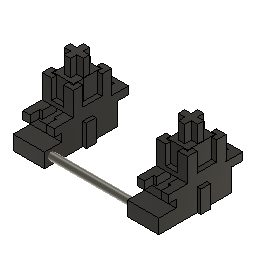
MX Cherry-style Stabilizer v10 (Autodesk Fusion 360 design; units mm, degrees)
Autodesk Fusion 360 part; units mm, degrees
note: some values were not read from the file. Chosen so that the rebuilt part matches the saved one: which bodies a step acts on; which face or edge a step refers to. Set by a fixed rule: which sketch regions a step uses.
sketch "Post Hole" plane through (0, 0, 0) normal (0, 0, 1) x (1, 0, 0)
  line L0 (-11.9, 5.93) -> (-7.7, 5.93)
  line L1 (-11.9, -7.57) -> (-10.4, -7.57)
  line L2 (1.75, 0) -> (22.5, 0)
  line L3 (-8.575, 2.3) -> (-7.7, 2.3)
  line L4 (-7.7, -0.5) -> (-7.7, 7.93)
  line L5 (-8.575, -0.5) -> (-7.7, -0.5)
  line L6 (-8.575, -0.5) -> (-8.575, -9.77)
  line L7 (-10.4, -6.77) -> (-8.575, -6.77)
  line L8 (-10.4, -8.27) -> (-10.4, -6.77)
  line L9 (-8.575, -9.77) -> (-11.9, -9.77)
  line L10 (-11.9, 9.93) -> (-8.575, 9.93)
  line L11 (-8.575, 9.93) -> (-8.575, 2.3)
  line L12 (-10.4, -8.27) -> (-11.9, -8.27)
  line L13 (-7.7, 7.93) -> (-11.9, 7.93)
  line L14 (-11.9, 11) -> (-11.9, -15.5609)
  line L15 (-10, -20) -> (13.8, -20)
  line L16 (-11.9, -7.57) -> (-13.4, -7.57)
  line L17 (-15.225, 9.93) -> (-15.225, 2.3)
  line L18 (-13.4, -8.27) -> (-13.4, -6.77)
  line L19 (-16.1, -0.5) -> (-16.1, 7.93)
  line L20 (-16.1, 7.93) -> (-11.9, 7.93)
  line L21 (-15.225, -0.5) -> (-16.1, -0.5)
  line L22 (-11.9, 5.93) -> (-16.1, 5.93)
  line L23 (-13.4, -6.77) -> (-15.225, -6.77)
  line L24 (-11.9, 9.93) -> (-15.225, 9.93)
  line L25 (-15.225, -0.5) -> (-15.225, -9.77)
  line L26 (-13.4, -8.27) -> (-11.9, -8.27)
  line L27 (-15.225, -9.77) -> (-11.9, -9.77)
  line L28 (-15.225, 2.3) -> (-16.1, 2.3)
  point P0 (-11.9, 11)
  dimension "d3" = 13.5
  dimension "d10" = 2
  dimension "d11" = 3
  dimension "d13" = 4
  dimension "d75" = 1.5
  dimension "d78" = 2.8
  dimension "d79" = 0.875
  dimension "d80" = 4.2
  dimension "d82" = 0.8
  dimension "d83" = 6.77
  dimension "d84" = 0.7
  dimension "d85" = 0.5
  dimension "ParameterA" = 23.8
  dimension "d87" = 11.9
  constraint coincident L14 L12.end
  constraint coincident L14 L1.start
  constraint coincident L14 L9.end
  constraint coincident L14 L0.start
  constraint coincident L14 L13.end
  constraint coincident L14 L10.start
  constraint coincident L4 L0.end
  constraint coincident L3.end L4
  constraint coincident L7.end L6
  constraint coincident L1.end L8
  constraint vertical L4
  constraint collinear L6 L11
  constraint horizontal L15
  constraint symmetric L1.end L14 L16.end
  constraint symmetric L3.start L14 L17.end
  constraint symmetric L3.end L14 L28.end
  constraint symmetric L4.start L14 L19.start
  constraint symmetric L5.start L14 L21.start
  constraint symmetric L7.end L14 L23.end
  constraint symmetric L7.start L14 L18.end
  constraint symmetric L6.end L14 L25.end
  constraint symmetric L10.end L14 L17.start
  constraint symmetric L8.start L14 L18.start
  constraint symmetric L4.end L14 L19.end
  constraint symmetric P0 L14 L14.start
  constraint symmetric L14 L12.end L26.end
  constraint symmetric L14 L1.start L16.start
  constraint symmetric L14 L9.end L27.end
  constraint symmetric L14 L13.end L20.end
  constraint symmetric L14 L10.start L24.start
  constraint symmetric L14 L0.start L22.start
  constraint symmetric L14 L0.end L22.end
  measures "d3" distance of L0 L1
  measures "d10" distance of L0 L13
  measures "d11" distance of L7 L9
  measures "d13" distance of L0 L10
  measures "d75" distance of L8 L14
  measures "d78" distance of L3 L5
  measures "d79" distance of L4 L6
  measures "d80" distance of L4 L14
  measures "d82" distance of L1 L7
  measures "d83" distance of L2 L7
  measures "d84" distance of L1 L12
  measures "d85" distance of L2 L5
  measures "ParameterA" distance of L15.start L15.end
  measures "d87" distance of origin L14
ref_plane "WorkPlane1" through (0, 0, -1.6) normal (0, 0, 1) x (1, 0, 0)
extrude "Extrude1" add sketch "Post Hole" along normal blind 10 contours L0 L11 L13 L14 | L14 L17 L20 L22 | L0 L1 L3 L4 L5 L6 L7 L8 L11 L14 | L14 L16 L17 L18 L19 L21 L22 L23 L25 L28 | L0 L4 L11 L13 | L0 L3 L4 L11 | L1 L8 L12 L14 | L14 L16 L18 L26 | L17 L19 L20 L22 | L17 L19 L22 L28 | L6 L7 L8 L9 L12 L14 | L14 L18 L23 L25 L26 L27 makes body 1
extrude "Extrude2" add sketch "Post Hole" against normal up to surface (1.6 mm away) separate body contours L0 L1 L3 L4 L5 L6 L7 L8 L11 L14 | L14 L16 L17 L18 L19 L21 L22 L23 L25 L28 makes body 2
extrude "Extrude3" add sketch "Post Hole" against normal blind 10 from surface at -1.6 separate body contours L0 L11 L13 L14 | L14 L17 L20 L22 | L0 L1 L3 L4 L5 L6 L7 L8 L11 L14 | L14 L16 L17 L18 L19 L21 L22 L23 L25 L28 | L10 L11 L13 L14 | L14 L17 L20 L24 | L1 L8 L12 L14 | L14 L16 L18 L26 makes body 3
sketch "Placeholder over Plate" plane through (0, 0, 0) normal (0, 0, 1) x (1, 0, 0)
  line L0 (1.75, 0) -> (22.5, 0)
  line L1 (-11.9, -7.5) -> (-8.65, -7.5)
  line L2 (20, 0) -> (2.5, 0)
  line L3 (-8.65, -4) -> (-11.9, -4)
  line L4 (-10.65, 4) -> (-10.65, 3)
  line L5 (-11.9, 3) -> (-9.65, 3)
  line L6 (-9.65, 2) -> (-8.65, 2)
  line L7 (-10.65, -3) -> (-9.65, -3)
  line L8 (-9.65, -3) -> (-9.65, 3)
  line L9 (-9.65, -2) -> (-8.65, -2)
  line L10 (-10.15, 8) -> (-10.15, 6)
  line L11 (-10.15, 6) -> (-10.65, 6)
  line L12 (-10.65, 6) -> (-10.65, 4)
  line L13 (-10.65, -3) -> (-10.65, -6.5)
  line L14 (-10.65, -6.5) -> (-11.9, -6.5)
  line L15 (-11.9, -5.2) -> (-8.65, -5.2)
  line L16 (-8.65, 0) -> (-7.9, 0)
  line L17 (-7.9, 0) -> (-7.9, 2)
  line L18 (-7.9, 2) -> (-8.65, 2)
  line L19 (-8.65, -7.5) -> (-8.65, 10)
  line L20 (-8.65, 10) -> (-11.9, 10)
  line L21 (-11.9, -10) -> (-11.9, 12)
  line L22 (-8.65, 4) -> (-11.9, 4)
  line L23 (-11.9, 6.4) -> (-8.65, 6.4)
  line L24 (-11.9, 8) -> (-8.65, 8)
  line L25 (-11.9, 6.4) -> (-15.15, 6.4)
  line L26 (-13.65, 6) -> (-13.15, 6)
  line L27 (-11.9, 3) -> (-14.15, 3)
  line L28 (-13.15, 4) -> (-13.15, 3)
  line L29 (-13.65, 8) -> (-13.65, 6)
  line L30 (-15.15, 10) -> (-11.9, 10)
  line L31 (-13.15, 6) -> (-13.15, 4)
  line L32 (-15.15, -7.5) -> (-15.15, 10)
  line L33 (-13.15, -6.5) -> (-11.9, -6.5)
  line L34 (-14.15, 2) -> (-15.15, 2)
  line L35 (-11.9, -5.2) -> (-15.15, -5.2)
  line L36 (-13.15, -3) -> (-13.15, -6.5)
  line L37 (-15.15, 0) -> (-15.9, 0)
  line L38 (-15.9, 0) -> (-15.9, 2)
  line L39 (-15.15, 4) -> (-11.9, 4)
  line L40 (-14.15, -2) -> (-15.15, -2)
  line L41 (-11.9, -7.5) -> (-15.15, -7.5)
  line L42 (-15.9, 2) -> (-15.15, 2)
  line L43 (-14.15, -3) -> (-14.15, 3)
  line L44 (-15.15, -4) -> (-11.9, -4)
  line L45 (-13.15, -3) -> (-14.15, -3)
  line L46 (-11.9, 8) -> (-15.15, 8)
  line L47 (-7.15, -9.5) -> (-16.65, -9.5)
  line L48 (-16.65, -9.5) -> (-16.65, 9.5)
  line L49 (-16.65, 9.5) -> (-7.15, 9.5)
  line L50 (-7.15, 9.5) -> (-7.15, -9.5)
  line L51 (-7.15, -9.5) -> (-16.65, 9.5) construction
  line L52 (-16.65, -9.5) -> (-7.15, 9.5) construction
  point P0 (-11.9, 12)
  point P1 (-11.9, -10)
  point P2 (-11.9, 0)
  dimension "d23" = 15.5
  dimension "d25" = 8
  dimension "d26" = 1
  dimension "d27" = 1
  dimension "d29" = 2
  dimension "d30" = 1.5
  dimension "d32" = 1
  dimension "d57" = 1.2
  dimension "d59" = 6
  dimension "d88" = 11.9
  dimension "d89" = 4
  dimension "d90" = 3.25
  dimension "d91" = 2
  dimension "d92" = 1.25
  dimension "d93" = 8
  dimension "d94" = 2.4
  dimension "d133" = 19
  dimension "d134" = 9.5
  constraint coincident L22.start L19
  constraint symmetric L22.start L2 L3.start
  constraint coincident L4.start L22
  constraint perpendicular L4 L22
  constraint perpendicular L4 L5
  constraint perpendicular L5 L8
  constraint coincident L6.end L19
  constraint perpendicular L6 L19
  constraint symmetric L2 L4.end L7.start
  constraint symmetric L2 L5.end L7.end
  constraint symmetric L2 L6.start L9.start
  constraint symmetric L2 L6.end L9.end
  constraint perpendicular L10 L11
  constraint perpendicular L11 L12
  constraint perpendicular L3 L13
  constraint perpendicular L13 L14
  constraint coincident L15.end L19
  constraint perpendicular L15 L19
  constraint coincident L23.end L19
  constraint coincident L16.start L19
  constraint perpendicular L16 L19
  constraint perpendicular L0 L17
  constraint perpendicular L19 L20
  constraint collinear L0 L16
  constraint perpendicular L17 L18
  constraint coincident L21 L1.start
  constraint coincident L21 L15.start
  constraint coincident L21 L3.end
  constraint coincident L21 L5.start
  constraint coincident L21 L22.end
  constraint coincident L21 L23.start
  constraint coincident L21 L24.start
  constraint coincident L24.end L19
  constraint coincident L4.end L5
  constraint coincident L6.start L8
  constraint coincident L14.end L21
  constraint coincident L10.start L24
  constraint symmetric L24.end L21 L46.end
  constraint symmetric L1.end L21 L32.start
  constraint symmetric L22.start L21 L39.start
  constraint symmetric L3.start L21 L44.start
  constraint symmetric L4.start L21 L28.start
  constraint symmetric L4.end L21 L28.end
  constraint symmetric L5.end L21 L27.end
  constraint symmetric L6.start L21 L34.start
  constraint symmetric L6.end L21 L34.end
  constraint symmetric L7.start L21 L36.start
  constraint symmetric L7.end L21 L43.start
  constraint symmetric L9.start L21 L40.start
  constraint symmetric L9.end L21 L40.end
  constraint symmetric L10.start L21 L29.start
  constraint symmetric L10.end L21 L26.start
  constraint symmetric L11.end L21 L26.end
  constraint symmetric L13.end L21 L33.start
  constraint symmetric L14.end L21 L33.end
  constraint symmetric L15.end L21 L35.end
  constraint symmetric L23.end L21 L25.end
  constraint symmetric L16.start L21 L37.start
  constraint symmetric L16.end L21 L37.end
  constraint symmetric L17.end L21 L38.end
  constraint symmetric L19.end L21 L30.start
  constraint symmetric L20.end L21 L30.end
  constraint symmetric P1 L21 L21.start
  constraint symmetric P0 L21 L21.end
  constraint symmetric L21 L1.start L41.start
  constraint symmetric L21 L15.start L35.start
  constraint symmetric L21 L3.end L44.end
  constraint symmetric L21 L5.start L27.start
  constraint symmetric L21 L22.end L39.end
  constraint symmetric L21 L23.start L25.start
  constraint symmetric L21 L24.start L46.start
  constraint horizontal L47
  constraint perpendicular L47 L48
  constraint parallel L47 L49
  constraint parallel L48 L50
  constraint coincident L51 P2
  constraint coincident L52 P2
  constraint coincident L21 P2
  constraint coincident L2 P2
  measures "d23" distance of L24.end L1.end
  measures "d25" distance of L3 L22
  measures "d26" distance of L5 L22
  measures "d27" distance of L8 L19
  measures "d29" distance of L6 L22
  measures "d30" distance of L10 L19
  measures "d32" distance of L1 L14
  measures "d57" distance of L3 L15
  measures "d59" distance of L20 L22
  measures "d88" distance of origin L21
  measures "d89" distance of L17 L21
  measures "d90" distance of L19 L21
  measures "d91" distance of L11 L24
  measures "d92" distance of L12 L21
  measures "d93" distance of origin L24
  measures "d94" distance of L22 L23
  measures "d133" distance of L47.end L48.end
  measures "d134" distance of L47.start L47.end
extrude "Extrude4" add sketch "Placeholder over Plate" along normal blind 1.6 separate body contours L1 L13 L14 L15 L19 L21 | L21 L32 L33 L35 L36 L41 | L3 L13 L15 L19 | L32 L35 L36 L44 | L10 L19 L23 L24 | L25 L29 L32 L46 | L10 L11 L12 L19 L22 L23 | L25 L26 L29 L31 L32 L39 makes body 4 at (-9.15, 6, 0) makes body 5 at (-14.65, 6, 0) makes body 6 at (-9.3167, -6, 0)
extrude "Extrude5" add sketch "Placeholder over Plate" along normal blind 6.5 contours L3 L7 L8 L9 L13 L19 | L32 L36 L40 L43 L44 L45 | L4 L5 L6 L8 L19 L22 | L27 L28 L32 L34 L39 L43 bodies 6 4 5
extrude "Extrude6" add sketch "Placeholder over Plate" along normal blind 2.5 contours L6 L8 L9 L19 | L32 L34 L40 L43 bodies 6 4 5
extrude "Extrude7" add sketch "Placeholder over Plate" along normal blind 0.9 from surface at 1.6 contours L4 L5 L21 L22 | L21 L27 L28 L39 | L4 L5 L6 L8 L19 L22 bodies 6
sketch "Placeholder Stem" plane through (0, 0, 6.5) normal (0, 0, 1) x (-1, 0, 0)
  line L0 (11.9, -4) -> (11.9, 0)
  line L1 (11.9, 0) -> (8.4, 0)
  line L2 (11.9, -2.8) -> (9.8, -2.8)
  line L3 (9.8, -2.8) -> (9.8, 0)
  line L4 (11.9, -0.65) -> (9.9, -0.65)
  line L5 (9.9, -0.65) -> (9.9, 0)
  line L6 (-1.75, 0) -> (-22.5, 0)
  line L7 (11.9, -2) -> (11.25, -2)
  line L8 (11.25, -2) -> (11.25, 0)
  line L9 (11.9, -0.65) -> (13.9, -0.65)
  line L10 (12.55, -2) -> (12.55, 0)
  line L11 (11.9, -2.8) -> (14, -2.8)
  line L12 (14, -2.8) -> (14, 0)
  line L13 (13.9, -0.65) -> (13.9, 0)
  line L14 (11.9, -2) -> (12.55, -2)
  line L15 (13.9, 0.65) -> (13.9, 0)
  line L16 (11.9, 2.8) -> (14, 2.8)
  line L17 (9.9, 0.65) -> (9.9, 0)
  line L18 (11.9, 2) -> (11.25, 2)
  line L19 (11.25, 2) -> (11.25, 0)
  line L20 (11.9, 2.8) -> (9.8, 2.8)
  line L21 (12.55, 2) -> (12.55, 0)
  line L22 (11.9, 0.65) -> (9.9, 0.65)
  line L23 (11.9, 0.65) -> (13.9, 0.65)
  line L24 (14, 2.8) -> (14, 0)
  line L25 (9.8, 2.8) -> (9.8, 0)
  line L26 (11.9, 2) -> (12.55, 2)
  point P0 (11.9, 0)
  point P1 (11.9, 0)
  point P2 (11.9, 0)
  dimension "d95" = 2.1
  dimension "d96" = 2.8
  dimension "d97" = 11.9
  dimension "d98" = 0.65
  dimension "d99" = 2
  dimension "d100" = 0.65
  dimension "d101" = 2
  constraint vertical L0
  constraint perpendicular L0 L1
  constraint coincident L0 L2.start
  constraint perpendicular L0 L2
  constraint coincident L1 L3.end
  constraint perpendicular L1 L3
  constraint coincident L0 L4.start
  constraint perpendicular L0 L4
  constraint coincident L1 L5.end
  constraint perpendicular L1 L5
  constraint collinear L1 L6
  constraint coincident L0 L7.start
  constraint perpendicular L0 L7
  constraint coincident L1 L8.end
  constraint perpendicular L1 L8
  constraint symmetric P1 L0 P0
  constraint symmetric L0 L2.start L11.start
  constraint symmetric L0 L2.end L11.end
  constraint symmetric L0 L3.end L12.end
  constraint symmetric L0 L4.start L9.start
  constraint symmetric L0 L4.end L9.end
  constraint symmetric L0 L5.end L13.end
  constraint symmetric L0 L7.start L14.start
  constraint symmetric L0 L7.end L10.start
  constraint symmetric L0 L8.end L10.end
  constraint symmetric P1 L1 P0
  constraint symmetric L1 L2.start L16.start
  constraint symmetric L1 L2.end L20.end
  constraint symmetric L1 L3.end L25.end
  constraint symmetric L1 L4.start L22.start
  constraint symmetric L1 L4.end L17.start
  constraint symmetric L1 L5.end L17.end
  constraint symmetric L1 L7.start L18.start
  constraint symmetric L1 L7.end L18.end
  constraint symmetric L1 L8.end L19.end
  constraint symmetric L1 P2 P1
  constraint symmetric L1 L10.start L21.start
  constraint symmetric L1 L10.end L21.end
  constraint symmetric L1 L11.end L16.end
  constraint symmetric L1 L9.end L15.start
  constraint symmetric L1 L12.end L24.end
  constraint symmetric L1 L13.end L15.end
  measures "d95" distance of L0 L3
  measures "d96" distance of L1 L2
  measures "d97" distance of origin L0
  measures "d98" distance of L1 L4
  measures "d99" distance of L0 L5
  measures "d100" distance of L0 L8
  measures "d101" distance of L1 L7
extrude "Extrude8" add sketch "Placeholder Stem" against normal blind 6 separate body contours L0 L1 L2 L3 L4 L5 L7 L8 | L0 L1 L9 L10 L11 L12 L13 L14 L15 L16 L17 L18 L19 L20 L21 L22 L23 L24 L25 L26 makes body 7
extrude "Extrude9" add sketch "Placeholder Stem" along normal blind 3.5 separate body contours L0 L4 L7 L8 | L0 L9 L10 L14 | L0 L1 L4 L8 | L0 L1 L9 L10 L19 L21 L22 L23 | L1 L4 L5 L8 | L9 L10 L13 L15 L21 L23 | L1 L17 L19 L22 | L18 L19 L21 L22 L23 L26 makes body 8
extrude "Extrude10" add sketch "Placeholder over Plate" against normal blind 1.6 separate body contours L3 L13 L15 L19 | L3 L13 L15 L21 | L21 L35 L36 L44 | L32 L35 L36 L44 | L3 L7 L8 L9 L13 L19 | L3 L5 L7 L8 L13 L21 | L21 L27 L36 L43 L44 L45 | L32 L36 L40 L43 L44 L45 | L6 L8 L9 L19 | L4 L5 L21 L22 | L21 L27 L28 L39 | L32 L34 L40 L43 | L16 L17 L18 L19 | L4 L5 L6 L8 L19 L22 | L21 L25 L26 L29 L31 L39 | L10 L11 L12 L21 L22 L23 | L27 L28 L32 L34 L39 L43 | L32 L37 L38 L42 | L10 L11 L12 L19 L22 L23 | L25 L26 L29 L31 L32 L39 makes body 9
extrude "Extrude11" add sketch "Placeholder over Plate" against normal blind 3 from surface at -1.6 separate body contours L13 L14 L15 L21 | L21 L33 L35 L36 | L3 L13 L15 L19 | L3 L13 L15 L21 | L21 L35 L36 L44 | L32 L35 L36 L44 | L3 L7 L8 L9 L13 L19 | L3 L5 L7 L8 L13 L21 | L21 L27 L36 L43 L44 L45 | L32 L36 L40 L43 L44 L45 | L6 L8 L9 L19 | L4 L5 L21 L22 | L21 L27 L28 L39 | L19 L20 L21 L49 | L19 L21 L24 L49 | L21 L32 L46 L49 | L21 L30 L32 L49 | L32 L34 L40 L43 | L16 L17 L18 L19 | L4 L5 L6 L8 L19 L22 | L21 L25 L26 L29 L31 L39 | L10 L11 L12 L21 L22 L23 | L27 L28 L32 L34 L39 L43 | L10 L19 L23 L24 | L25 L29 L32 L46 | L32 L37 L38 L42 | L10 L11 L12 L19 L22 L23 | L21 L25 L29 L46 | L10 L21 L23 L24 | L25 L26 L29 L31 L32 L39 makes body 10
move_body "Move1" bodies 6 7 8 9 10 to x (1, 0, 0) y (0, 1, 0) z (0, 0, 1) at (0, -0.5, 0)
combine "Combine1" operation add target body 7 tool bodies 8
combine "Combine2" operation add target body 6 tool bodies 9
copy_body "CopyPasteBodies1" bodies 6 makes body 11
combine "Combine3" operation add target body 11 tool bodies 10 keep tools
combine "Combine4" operation add target body 1 tool bodies 2 3
fillet "Fillet2" radius 0.1 72 edges at (-11.9, 9.93, -11.6) (-11.9, 9.93, -1.6) (-15.225, 4.115, 0) (-16.1, 3.715, 10) (-8.1375, 2.3, 0) (-8.575, 4.115, 0) (-15.6625, -0.5, -11.6) (-7.7, 3.715, 10) (-14.3125, -6.77, 0) (-8.575, -8.27, 0) (-7.7, 5.115, 0) (-11.9, 5.93, -1.6) (-16.1, 5.115, 0) (-10.4, -8.27, -6.6) (-15.225, 2.3, -5.8) (-15.225, -9.77, 5) (-9.4875, -6.77, -11.6) (-8.575, 6.115, -11.6) (-13.4, -7.92, -1.6) (-15.225, -0.5, -0.8) (-10.4, -7.52, -11.6) (-11.9, -8.27, -11.6) (-15.6625, 2.3, 0) (-13.4, -7.17, 0) (-11.9, -9.77, 0) (-15.225, -5.135, 10) (-8.575, -0.5, -0.8) (-16.1, -0.5, -0.8) (-8.575, -3.635, -11.6) (-15.225, -6.77, -5.8) (-13.4, -6.77, -5.8) (-7.7, -0.5, -0.8) (-8.575, 5.93, -0.8) (-13.4, -7.57, -0.8) (-10.4, -7.57, -0.8) (-8.575, -5.135, 10) (-15.225, -3.635, -11.6) (-7.7, 2.3, -5.8) (-10.4, -6.77, -5.8) (-8.575, -6.77, -5.8) (-16.1, 2.3, -5.8) (-15.6625, -0.5, 10) (-11.9, -7.57, 0) (-11.9, 7.93, 10) (-16.1, 0.9, -11.6) (-11.9, 5.93, 0) (-15.6625, 2.3, -11.6) (-8.575, 9.93, -6.6) (-15.225, -8.27, 0) (-9.4875, -6.77, 0) (-8.1375, -0.5, 10) (-8.1375, -0.5, -11.6) (-15.225, 9.93, -6.6) (-11.9, -9.77, 10) (-8.1375, 2.3, -11.6) (-11.9, 7.93, 0) (-10.4, -7.17, 0) (-8.575, 7.93, -1.6) (-8.575, -9.77, 5) (-7.7, 0.9, -11.6) (-15.225, 6.115, -11.6) (-15.225, 7.93, -1.6) (-11.9, -7.57, -1.6) (-11.9, -8.27, -1.6) (-13.4, -7.52, -11.6) (-16.1, 7.93, 5) (-7.7, 7.93, 5) (-14.3125, -6.77, -11.6) (-10.4, -7.92, -1.6) (-13.4, -8.27, -6.6) (-8.575, 2.3, -5.8) (-15.225, 5.93, -0.8) 26 faces at (-15.225, 6.0533, -8.2667) (-7.7, 3.2433, 6.6667) (-13.4, -7.5367, -8.2667) (-8.2833, 2.3, -3.8667) (-10.4, -7.5367, -8.2667) (-9.7917, -6.77, -3.8667) (-15.5167, 2.3, -3.8667) (-8.2833, -0.5, 2.8) (-15.5167, -0.5, 2.8) (-14.0083, -6.77, -3.8667) (-11.4, -7.57, -0.5333) (-8.575, -5.68, 6.6667) (-16.1, 3.2433, 6.6667) (-10.7917, 7.2633, -1.6) (-10.5, 7.93, 3.3333) (-11.4, -9.0367, 0) (-13.0083, 7.2633, 0) (-13.0083, -9.77, 3.3333) (-12.4, -7.8033, -1.6) (-12.4, -8.27, -4.9333) (-13.0083, 5.12, 10) (-10.7917, 9.93, -4.9333) (-13.0083, 7.3867, -11.6) (-15.225, -5.68, 6.6667) (-13.0083, 5.93, -0.5333) (-8.575, 6.0533, -8.2667) on bodies 1
fillet "Fillet3" radius 0.1 180 edges at (-15.15, -0.5, 2.5) (-10.65, -3.5, 3.25) (-15.15, -8, 0.8) (-9.65, -0.5, 0) (-7.9, 0.5, -4.6) (-13.15, -7, 0.8) (-11.9, -7, 1.6) (-9.65, 2.5, 3.25) (-8.65, -8, 0.8) (-9.65, -3.5, 3.25) (-14.15, -0.5, 2.5) (-14.15, -0.5, 0) (-15.15, 0.5, 0) (-7.9, 0.5, 0) (-8.65, -0.5, 2.5) (-14.15, -5.7, -4.6) (-10.65, -5.75, 1.6) (-15.15, 5.5, -4.6) (-15.15, -6.25, 1.6) (-8.65, -6.25, 1.6) (-11.9, 2.5, 2.5) (-15.9, 0.5, 0) (-15.9, 0.5, -4.6) (-8.65, 0.5, 0) (-9.65, -0.5, 2.5) (-10.65, -5.7, -3.1) (-15.525, -0.5, 0) (-10.4, 5.5, 1.6) (-13.65, 6.5, 1.6) (-7.9, -0.5, -2.3) (-8.65, 7.5, 0.8) (-10.15, 6.7, 0) (-15.15, 6.7, 0) (-11.9, -7, 0) (-8.275, -0.5, -4.6) (-11.9, -5.7, 0) (-10.65, -7, -3.1) (-13.15, 2.5, 0.8) (-10.15, 6.5, 1.6) (-10.15, -3.5, 0) (-10.15, 5.5, 0.8) (-10.65, -6.35, -1.6) (-9.65, 3.5, 1.6) (-14.4, 7.5, 1.6) (-13.15, -6.35, -1.6) (-13.65, 7.5, 0.8) (-13.15, 5.5, 0.8) (-14.15, 3.5, 1.6) (-10.65, 2.5, 0.8) (-13.15, 3, 1.6) (-15.9, -0.5, -2.3) (-8.65, 6.7, 0) (-13.15, -4.5, 4.05) (-14.65, -2.5, 6.5) (-10.65, -4, 6.5) (-13.15, -4.6, 0) (-8.65, 1.5, -2.3) (-11.9, 5.9, 0) (-11.9, 3.5, 1.6) (-11.9, 9.5, -1.6) (-10.65, 3, 6.5) (-9.65, 3.5, 6.5) (-11.9, 5.9, -1.6) (-15.15, 1.5, -2.3) (-7.9, 1.5, -2.3) (-13.65, -3.5, 0) (-10.65, -6.35, -4.6) (-14.15, -4.5, 1.6) (-10.15, -3.5, 6.5) (-11.9, -7, -1.6) (-13.15, 3, 6.5) (-14.15, -3, 6.5) (-9.65, 2, 6.5) (-14.15, 3.5, 6.5) (-14.65, -2.5, 2.5) (-8.65, 2.5, 6.5) (-15.15, -3.1, -4.6) (-15.15, 2.5, 6.5) (-9.65, -3, 6.5) (-11.9, 2.5, 1.6) (-13.15, -4, 6.5) (-8.65, -6.85, 0) (-14.15, -2.5, 4.5) (-10.65, 3.5, 4.5) (-9.65, -4.5, 6.5) (-13.15, 4.5, 1.6) (-10.15, 2.5, 6.5) (-10.65, -4.6, 0) (-15.15, -3.5, 6.5) (-15.15, -2.5, 4.5) (-10.65, 3, 2.5) (-14.15, 1.5, 4.5) (-9.15, 1.5, 2.5) (-14.65, 1.5, 2.5) (-9.15, -2.5, 6.5) (-9.65, -4.5, 1.6) (-9.15, -2.5, 2.5) (-8.65, -3.5, 6.5) (-9.15, 1.5, 6.5) (-13.15, 3, 2.5) (-15.15, 1.5, 4.5) (-13.65, 2.5, 6.5) (-8.65, -3.1, -4.6) (-14.65, 1.5, 6.5) (-15.15, 5.5, 1.6) (-11.9, 9.5, -4.6) (-10.65, -7, 0.8) (-13.15, -3.5, 3.25) (-14.15, -3.5, 3.25) (-15.15, 3.5, 4.05) (-13.15, 3.5, 4.5) (-8.65, 5.5, -4.6) (-9.65, -2.5, 4.5) (-11.9, 3.5, 2.5) (-8.65, -5.7, -2.3) (-13.15, 4, 0) (-10.65, -4.5, 4.05) (-9.65, -5.7, -4.6) (-8.65, 1.5, 4.5) (-13.15, -5.75, 1.6) (-14.15, -4.5, 6.5) (-10.65, 2.5, 4.5) (-8.65, 5.5, 1.6) (-10.65, 4.5, 1.6) (-15.15, -6.85, 0) (-8.65, -2.5, 4.5) (-9.65, -5.7, 0) (-14.15, -5.7, 0) (-15.15, -4.5, 4.05) (-13.15, 2.5, 4.5) (-10.65, 4, 0) (-9.65, 1.5, 4.5) (-8.65, -4.5, 4.05) (-13.65, -3.5, 6.5) (-8.65, 3.5, 4.05) (-15.15, -5.7, -2.3) (-14.15, 2.5, 3.25) (-11.9, -8, 1.6) (-13.65, 6.7, 0) (-9.4, 5.9, 0) (-15.15, 7.7, -1.6) (-15.525, -0.5, -4.6) (-8.275, -0.5, 0) (-10.15, 2.5, 0) (-8.275, 1.5, -4.6) (-15.15, -0.5, -2.3) (-15.525, 1.5, 0) (-13.65, 2.5, 0) (-9.4, 7.5, 0) (-10.65, 3, 1.6) (-14.15, 2, 6.5) (-13.15, -6.35, 0) (-15.15, 9.5, -3.1) (-8.65, 9.5, -3.1) (-8.275, 1.5, 0) (-8.65, -0.5, -2.3) (-10.65, -6.35, 0) (-15.9, 1.5, -2.3) (-8.65, 7.7, -1.6) (-9.4, 7.5, 1.6) (-13.15, -5.7, -3.1) (-8.65, 5.9, -0.8) (-15.15, 5.9, -0.8) (-15.525, 1.5, -4.6) (-13.65, 5.5, 0.8) (-13.4, 5.5, 0) (-13.15, -7, -3.1) (-10.15, 7.5, 0.8) (-13.4, 5.5, 1.6) (-13.65, 5.7, 0) (-11.9, -7, -4.6) (-14.4, 7.5, 0) (-10.4, 5.5, 0) (-14.4, 5.9, 0) (-15.15, 7.5, 0.8) (-10.15, 5.7, 0) (-13.15, -6.35, -4.6) (-11.9, -8, 0) (-11.9, -5.7, -1.6) (-10.65, 5.5, 0.8) 60 faces at (-8.65, -3.9667, -1.5333) (-9.65, -1.1667, 0.8333) (-12.3167, -6.5667, -1.6) (-10.65, -5.7333, 1.0667) (-9.65, 7.5, 0.5333) (-13.65, 6.3, 1.0667) (-14.15, 7.5, 0.5333) (-12.3167, -7, -2.6) (-13.15, 3.8333, 0.5333) (-13.4833, 5.5, 0.5333) (-15.65, 1.5, -1.5333) (-10.8167, 7.1, -1.6) (-14.65, 5.5, 1.6) (-9.15, 5.5, 1.6) (-12.3167, 2.8333, 1.6) (-9.65, -4.1667, 6.5) (-8.4, -0.5, -1.5333) (-15.65, -0.5, -3.0667) (-12.3167, 2.8333, 2.5) (-10.65, 3.8333, 0.5333) (-11.4833, -7, 0.5333) (-13.4833, -3.5, 2.1667) (-10.3167, 5.5, 0.5333) (-14.4833, -1.1667, 2.5) (-10.3167, -3.5, 2.1667) (-13.8167, 2.5, 3) (-10.8167, -8, 0.5333) (-8.4, 0.8333, 0) (-9.15, 6.4333, 0) (-10.65, 3.1667, 3.8333) (-14.15, 6.9667, 0) (-13.15, 3.1667, 3.8333) (-14.4833, -4.5, 3.2333) (-14.15, -4.1667, 6.5) (-14.15, -1.1667, 0.8333) (-12.9833, 4.1667, -4.6) (-13.15, -5.7333, 1.0667) (-15.15, -3.9667, -1.5333) (-11.4833, -1.5, 0) (-8.9833, -1.1667, 2.5) (-10.8167, 9.5, -2.6) (-9.3167, -6.9, 0) (-9.3167, -5.7, -2.0667) (-13.15, -6.1333, -2.6) (-14.4833, 3.5, 3.5333) (-7.9, 0.1667, -1.5333) (-10.15, 6.3, 1.0667) (-10.65, -6.1333, -2.6) (-9.3167, -6.5, 1.6) (-9.65, 3.1667, 6.5) (-15.9, 0.1667, -1.5333) (-11.3167, 5.9, -1.0667) (-8.4, 1.5, -3.0667) (-9.3167, -2.5, 3.8333) (-14.15, 3.1667, 6.5) (-14.4833, 1.5, 3.8333) (-9.3167, -4.5, 3.2333) (-14.4833, -2.5, 3.8333) (-9.3167, 1.5, 3.8333) (-15.65, 0.1667, 0) on bodies 11
ref_plane "WorkPlane2" through (0, 0, -3) normal (0, 0, 1) x (1, 0, 0)
sketch "Sketch8" plane through (0, 0, -3) normal (0, 0, 1) x (1, 0, 0)
  line L0 (0, 8) -> (-11.9, 8)
  line L1 (0, 2.5) -> (0, 20)
  line L2 (0, 8) -> (11.9, 8)
  dimension "d109" = 11.9
  dimension "d110" = 8
  constraint horizontal L0
  constraint symmetric L0.start L1 L2.start
  constraint symmetric L0.end L1 L2.end
  measures "d109" distance of L0.start L0.end
  measures "d110" distance of origin L0
pipe "Pipe2" add diameter 1.5 path "Sketch8" along L0 L2 separate body makes body 12
extrude "Extrude15" add sketch "Placeholder over Plate" along normal blind 2 and the other way blind 2 separate body contours L1 L13 L14 L15 L19 L21 | L21 L32 L33 L35 L36 L41 | L1 L16 L17 L18 L19 L21 L47 L49 L50 | L21 L32 L37 L38 L41 L42 L47 L48 L49 | L13 L14 L15 L21 | L21 L33 L35 L36 | L3 L13 L15 L19 | L3 L13 L15 L21 | L21 L35 L36 L44 | L32 L35 L36 L44 | L3 L7 L8 L9 L13 L19 | L3 L5 L7 L8 L13 L21 | L21 L27 L36 L43 L44 L45 | L32 L36 L40 L43 L44 L45 | L6 L8 L9 L19 | L4 L5 L21 L22 | L21 L27 L28 L39 | L19 L21 L24 L49 | L21 L32 L46 L49 | L32 L34 L40 L43 | L16 L17 L18 L19 | L4 L5 L6 L8 L19 L22 | L21 L25 L26 L29 L31 L39 | L10 L11 L12 L21 L22 L23 | L27 L28 L32 L34 L39 L43 | L10 L19 L23 L24 | L25 L29 L32 L46 | L32 L37 L38 L42 | L10 L11 L12 L19 L22 L23 | L21 L25 L29 L46 | L10 L21 L23 L24 | L25 L26 L29 L31 L32 L39 makes body 13
mirror "Mirror1" about plane through (0, 0, 0) normal (1, 0, 0) of bodies 1 6 7 10 11 makes body 14 at (8.575, -5.6985, 6.6317) makes body 15 at (9.8, -1.4333, 4.5) makes body 16 at (11.9, 7.1, -1.6) makes body 17 at (10.8167, -3.9667, -1.6) makes body 18 at (10.85, 4.2, -4.6)
mirror "Mirror2" about plane through (0, 0, 0) normal (1, 0, 0) of bodies 13 makes body 19
sketch "Sketch9" plane through (0, 0, 0) normal (1, 0, 0) x (0, 1, 0)
  circle A0 centre (8, -3) radius 1
  line L0 (1.75, 0) -> (22.5, 0)
  circle A1 centre (5, -3) radius 1
  line L1 (4, -12) -> (4, -3)
  line L2 (6, -12) -> (6, -3)
  line L3 (4, -12) -> (6, -12)
  line L4 (8, -2) -> (5, -2)
  line L5 (8.0005, -4) -> (5, -4)
  dimension "d117" = 2
  dimension "d118" = 3
  dimension "d119" = 8
  dimension "d120" = 2
  dimension "d121" = 3
  dimension "d122" = 3
  dimension "d123" = 9
  constraint coincident A1 L1.end
  constraint tangent A1 L1
  constraint coincident A1 L2.end
  constraint tangent A1 L2
  constraint perpendicular L1 L3
  constraint perpendicular L2 L3
  constraint vertical L1
  constraint perpendicular L1 L4
  constraint horizontal L5
  constraint coincident A1 L5.end
  constraint coincident A0 L5.start
  constraint coincident A0 L4.start
  constraint coincident A1 L4.end
  constraint tangent A1 L5
  constraint tangent A1 L4
  measures "d117" diameter of A0
  measures "d118" distance of A0.centre L0
  measures "d119" horizontal distance of origin A0.centre
  measures "d120" diameter of A1
  measures "d121" distance of A0.centre A1.centre
  measures "d122" distance of L0 A1.centre
  measures "d123" distance of L1.start L1.end
extrude "Extrude14" add sketch "Sketch9" along normal up to surface (-11.9 mm away) and the other way up to surface (-11.9 mm away) separate body makes body 20
copy_body "CopyPasteBodies2" bodies 20 makes body 21
combine "Combine7" operation add target body 1 tool bodies 14 20
combine "Combine8" operation add target body 11 tool bodies 18 21
combine "Combine9" operation add target body 6 tool bodies 7 10 16 15 17 makes body 24 at (12.9833, 4.1667, -4.6) makes body 23 at (-9.8, -1.4333, 4.5) makes body 23 at (-11.6833, -1.6, 6.5) makes body 22 at (9.8, -1.4333, 4.5) makes body 22 at (11.6833, -1.6, 6.5)
copy_body "CopyPasteBodies3" bodies 1 makes body 25
move_body "Move2" bodies 25 11 24 23 22 6 12 1 to x (-1, 0, 0) y (0, -1, 0) z (0, 0, 1) at (0, 0, 0)
move_body "Move3" bodies 1 6 12 22 23 24 11 13 19 25 to x (1, 0, 0) y (0, 1, 0) z (0, 0, 1) at (0, 0, 0)
move_body "Move4" bodies 1 6 12 22 23 24 11 13 19 25 to x (1, 0, 0) y (0, 1, 0) z (0, 0, 1) at (0, 0, 0)
hidden bodies 25 1 11 13 19
equation "d87 = ParameterA / 2"
equation "d88 = ParameterA / 2"
equation "d97 = ParameterA / 2"
equation "d109 = ParameterA / 2"
equation "SwitchAngle = 0.0 deg"
equation "SwitchX = 0.00 mm"
equation "SwitchY = 0.00 mm"
named bodies: "Hole (1)", "MEV (1)", "Wire", "Territory"
